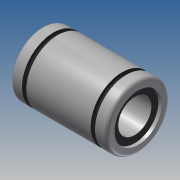
# Autodesk Inventor part: LM10UU
Saved by Autodesk Inventor 2015 SP1 (Build 190203100, 203)
## iProperties
Created: 2014-01-11
Part Number: LM10UU
Material: Generico
Document SubType Name: Modeling
Designer: Matteo
Density: 1 g/cm^3
Appearance: Stahl
Author: Matteo
Autodesk Inventor part; units mm, degrees
ref_plane "YZ Plane" through (0, 0, 0) normal (1, 0, 0) x (0, 1, 0)
ref_plane "XZ Plane" through (0, 0, 0) normal (0, 1, 0) x (-1, 0, 0)
ref_plane "XY Plane" through (0, 0, 0) normal (0, 0, 1) x (1, 0, 0)
sketch "Schizzo1" plane through (0, 0, 0) normal (0, 1, 0) x (-1, 0, 0)
  line L0 (-14.5, 5) -> (-14.5, 9.5)
  line L1 (-14.5, 9.5) -> (-11, 9.5)
  line L2 (-11, 9.5) -> (-11, 8.5)
  line L3 (-11, 8.5) -> (-9.7, 8.5)
  line L4 (-9.7, 8.5) -> (-9.7, 9.5)
  line L5 (-9.7, 9.5) -> (0, 9.5)
  line L6 (0, 9.5) -> (0, 5)
  line L7 (0, 5) -> (-14.5, 5)
  line L8 (0, 0) -> (5.7518, 0)
  dimension "d0" = 10
  dimension "d2" = 19
  dimension "d3" = 14.5
  dimension "d4" = 11
  dimension "d5" = 1.3
  dimension "d6" = 17
  constraints: 18 end point, 6 parallel, 1 collinear, 1 horizontal alignment, 1 perpendicular, 1 vertical, 1 vertical alignment
  measures "d0" diameter of L7 L8
  measures "d2" diameter of L5 L8
  measures "d3" distance between parallel lines of L6 L0
  measures "d4" distance from line of L6 L1.end
  measures "d5" distance of L2.end L3.end
  measures "d6" diameter of L3 L8
revolve "Rivoluzione1" add sketch "Schizzo1" angle 360 about axis through (0, 0, 0) along (-1, 0, 0)
fillet "Raccordo1" radius 1 1 edges at (14.5, 0, -9.5)
sketch "Schizzo2" plane through (14.5, 0, 0) normal (1, 0, 0) x (0, 0, -1)
  circle A0 centre (0, 0) radius 8.5 projected
  circle A1 centre (0, 0) radius 7.1007
  constraints: 1 centre point, 1 coincident
extrude "Estrusione2" cut sketch "Schizzo2" against normal blind 1 contours A1
mirror "Specchio1" about plane through (0, 0, 7.25) normal (-1, 0, 0)
